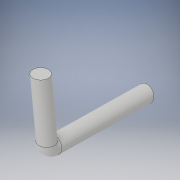
# Autodesk Inventor part: ACL_femur_hole
Saved by Autodesk Inventor 2019 (Build 230136000, 136)
## iProperties
Created: 2018-09-12
Part Number: ACL_femur_hole
Material: Generic
Document SubType Name: Modeling
Designer: HIVE
Density: 1 g/cm^3
Appearance: Default
Author: HIVE
Autodesk Inventor part; units mm, degrees
ref_plane "YZ Plane" through (0, 0, 0) normal (1, 0, 0) x (0, 1, 0)
ref_plane "XZ Plane" through (0, 0, 0) normal (0, 1, 0) x (-1, 0, 0)
ref_plane "XY Plane" through (0, 0, 0) normal (0, 0, 1) x (1, 0, 0)
sketch "Sketch1" plane through (0, 0, 0) normal (0, 1, 0) x (-1, 0, 0)
  circle A0 centre (0, 0) radius 2.5
  dimension "d0" = 5
  constraints: 1 centre point, 1 coincident
  measures "d0" diameter of A0
sketch "Sketch3" plane through (0, 0, 0) normal (1, 0, 0) x (0, 1, 0)
  line L0 (0, 0) -> (-20, -1.957)
  arc A0 (-20, -1.957) -> (-22.2293, -4.3746) centre (-19.7594, -4.4154) ccw
  line L1 (-22.2293, -4.3746) -> (-22.7252, -34.3746)
  line L2 (-27.2702, 0) -> (4.545, 0) projected
  dimension "d1" = 20
  dimension "d2" = 2.4702
  dimension "d3" = 96.535
  dimension "d4" = 5.589
  dimension "d5" = 30
  constraints: 4 end point, 2 point on circle, 2 tangent, 1 centre point
  measures "d1" horizontal distance of L0.start L0.end
  measures "d2" radius of A0
  measures "d3" angle of L0 L1
  measures "d4" angle of L0 L2
  measures "d5" vertical distance of L1.start L1.end
sweep "Sweep1" add profiles "Sketch1" path "Sketch3" path curves L0 A0 L1
body "Solid1"
